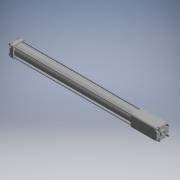
# Autodesk Inventor part: CE263-800(0)_BODY
Saved by Autodesk Inventor 2017.3 (Build 213256000, 256)
## iProperties
Part Number: CE263-800(0)_BODY
Material: Generic
Catalog Web Link: www.cadenas.de
Description: CE2 BODY-Stroke Reading Cylinder with Brake
Vendor: SMC
Document SubType Name: Modeling
Designer: partserver
Manufacturer: SMC
Mass: 2570.06 g
Surface Area: 5697.47 cm^2
Volume: 2570.06 cm^3
Density: 1 g/cm^3
Appearance: PSOLRGB-192-192-192
Category: PARTsolutions
Company: SMC
Title: CE263-800_BODY
Author: Cadenas PARTsolutions
Comments: Stroke Reading Cylinder with Brake
PSOL_IDENT_0: {$CADENAS_DATA\23d-libs\smc_jp\actuator\stroke_reading_cylinders\ce2\parts\ce2_body.prj},202 {VTYP=3
PSOL_IDENT_1: D},{NB=CE263-800(0)_BODY},{LINA=CE263-800_BODY},{NN=CE2 BODY},{DATE=05.07.2021 01:49:16},{GEOMDATE=2
PSOL_IDENT_2: 7.03.2020 05:40:07},{VERSION=},{LINEID=150},{WBVAR=THREAD1,STROKE,THREAD2},{WBNUMERIC=STROKE}  {NB=C
PSOL_IDENT_3: E263-800(0)_BODY},{LINA=CE263-800_BODY},{KT=DUMMY},{ORDER=CE263-800},{BORE=63},{THREAD1=},{STROKE=80
PSOL_IDENT_4: 0},{THREAD2=0},{A=35.000},{AA=60.000},{AL=32.000},{BB=98.500},{BL=27.000},{B=85.000},{C=48.500},{CC=
PSOL_IDENT_5: 23.000},{C1=64.000},{DD=24.000},{D=20.000},{EF=28.500},{EE=13.500},{E=40.000},{F=10.000},{FF=15.000}
PSOL_IDENT_6: ,{GA=174.000},{GB=17.000},{GC=26.000},{GD=67.000},{GL=18.000},{H1=11.000},{J=M10x1.25},{JRA=10.000},
PSOL_IDENT_7: {JRP=1.250},{K=9.000},{M=14.000},{MM=M18x1.5},{MMRA=18.000},{N=31.000},{NN=187.000},{P=3/8},{PND=16.
PSOL_IDENT_8: 662},{PH=11.700},{S=254.000},{W=0.000},{L1=22.000},{L2=73.000},{L3=72.000},{L4=9.100},{L5=5.300},{L6=
PSOL_IDENT_9: 35.000},{L7=13.000},{L8=9.500},{L9=14.000},{L10=9.200},{L11=9.200},{L12=2.500},{L13=9.000},{L14=48.5
PSOL_IDENT_10: 00},{L15=60.000},{LL1=23.000},{LL2=5.000},{LL3=6.000},{LL4=15.000},{LL5=8.000},{LL6=5.130},{LL7=4.50
PSOL_IDENT_11: 0},{LL8=38.500},{LL9=12.500},{LL0=109.500},{LL10=28.500},{L16=4.300},{L17=6.000},{L18=10.600},{L19=9
PSOL_IDENT_12: .820},{L20=10.500},{ZT=263.000},{H=58.000},{OFFET=18},{FONT=9}
NB: CE263-800(0)_BODY
NN: 187
NT: Stroke Reading Cylinder with Brake
NBSYN: $ORDER.($THREAD2.)_BODY
LINA: CE263-800_BODY
CATALOG: SMC (JP
BORE: 63
THREAD1: (-) Rc
STROKE: 800
THREAD2: on
A: 35
AA: 60
AL: 32
BB: 98.5
BL: 27
B: 85
C: 48.5
CC: 23
C1: 64
DD: 24
D: 20
EF: 28.5
EE: 13.5
E: 40
F: 10
FF: 15
GA: 174
GB: 17
GC: 26
GD: 67
GL: 18
H1: 11
J: M10x1.25
JRA: 10
JRP: 1.25
K: 9
M: 14
MM: M18x1.5
MMRA: 18
N: 31
P: 3/8
PND: 16.662
PH: 11.7
S: 254
W: 0
L1: 22
L2: 73
L3: 72
L4: 9.1
L5: 5.3
L6: 35
L7: 13
L8: 9.5
L9: 14
L10: 9.2
L11: 9.2
L12: 2.5
L13: 9
L14: 48.5
L15: 60
LL1: 23
LL2: 5
LL3: 6
LL4: 15
LL5: 8
LL6: 5.13
LL7: 4.5
LL8: 38.5
LL9: 12.5
LL0: 109.5
LL10: 28.5
L16: 4.3
L17: 6
L18: 10.6
L19: 9.82
L20: 10.5
ZT: 263
H: 58
SUPPLIER: SMC
ARTICLENO: CE263-800(0)_BODY
BOMINFO: CE263-800_BODY
CREATOR: CADENAS GmbH
Autodesk Inventor part; units mm, degrees
sketch "Sketch_1" plane through (0, 0, 0) normal (1, 0, 0) x (0, 1, 0)
  line L0 (31.5, 42.5) -> (-31.5, 42.5)
  arc A0 (-31.5, 42.5) -> (-42.5, 31.5) centre (-31.5, 31.5) ccw
  line L1 (-42.5, 31.5) -> (-42.5, -31.5)
  arc A1 (-42.5, -31.5) -> (-31.5, -42.5) centre (-31.5, -31.5) ccw
  line L2 (-31.5, -42.5) -> (31.5, -42.5)
  arc A2 (31.5, -42.5) -> (42.5, -31.5) centre (31.5, -31.5) ccw
  line L3 (42.5, -31.5) -> (42.5, 31.5)
  arc A3 (42.5, 31.5) -> (31.5, 42.5) centre (31.5, 31.5) ccw
  constraints: 8 end point, 8 point on circle, 4 centre point
extrude "Extrusion1" add sketch "Sketch_1" along normal blind 185.4
sketch "Sketch_2" plane through (0, 0, 0) normal (0, 0, 1) x (1, 0, 0)
  line L0 (187, 0) -> (185.4, 0)
  line L1 (185.4, 0) -> (185.4, 36.5)
  line L2 (185.4, 36.5) -> (187, 36.5)
  line L3 (187, 36.5) -> (187, 0)
  line L4 (187, 0) -> (185.4, 0)
  constraints: 10 end point
revolve "Revolution1" add sketch "Sketch_2" angle 360 about axis through (187, 0, 0) along (1, 0, 0)
sketch "Sketch_3" plane through (0, 0, 0) normal (0, 0, 1) x (1, 0, 0)
  line L0 (1023, 0) -> (187, 0)
  line L1 (187, 0) -> (187, 36)
  line L2 (187, 36) -> (1023, 36)
  line L3 (1023, 36) -> (1023, 0)
  line L4 (1023, 0) -> (187, 0)
  constraints: 10 end point
revolve "Revolution2" add sketch "Sketch_3" angle 360 about axis through (1023, 0, 0) along (1, 0, 0)
sketch "Sketch_41" plane through (0, 0, 0) normal (0, 0, 1) x (1, 0, 0)
  line L0 (1028.3, 0) -> (1023, 0)
  line L1 (1023, 0) -> (1023, 36.5)
  line L2 (1023, 36.5) -> (1028.3, 36.5)
  line L3 (1028.3, 36.5) -> (1028.3, 0)
  line L4 (1028.3, 0) -> (1023, 0)
  constraints: 10 end point
revolve "Revolution3" add sketch "Sketch_41" angle 360 about axis through (1028.3, 0, 0) along (1, 0, 0)
sketch "Sketch_4" plane through (1028.3, 0, 0) normal (1, 0, 0) x (0, 0, -1)
  line L0 (-42.5, 31.5) -> (-42.5, -31.5)
  arc A0 (-42.5, -31.5) -> (-31.5, -42.5) centre (-31.5, -31.5) ccw
  line L1 (-31.5, -42.5) -> (31.5, -42.5)
  arc A1 (31.5, -42.5) -> (42.5, -31.5) centre (31.5, -31.5) ccw
  line L2 (42.5, -31.5) -> (42.5, 31.5)
  arc A2 (42.5, 31.5) -> (31.5, 42.5) centre (31.5, 31.5) ccw
  line L3 (31.5, 42.5) -> (-31.5, 42.5)
  arc A3 (-31.5, 42.5) -> (-42.5, 31.5) centre (-31.5, 31.5) ccw
  constraints: 8 end point, 8 point on circle, 4 centre point
extrude "Extrusion2" add sketch "Sketch_4" along normal blind 25.7
sketch "Sketch_5" plane through (0, 42.5, 0) normal (0, 1, 0) x (1, 0, 0)
  line L0 (1024, 17.5) -> (1024, -17.5)
  line L1 (1024, -17.5) -> (1028.3, -19.9826)
  line L2 (1028.3, -19.9826) -> (1028.3, 19.9826)
  line L3 (1028.3, 19.9826) -> (1024, 17.5)
  constraints: 8 end point
extrude "Extrusion3" add sketch "Sketch_5" against normal blind 42.5
sketch "Sketch_11" plane through (0, 0, 0) normal (1, 0, 0) x (0, 1, 0)
  line L0 (-44.5, 44.5) -> (-44.5, -44.5)
  line L1 (-44.5, -44.5) -> (44.5, -44.5)
  line L2 (44.5, -44.5) -> (44.5, 44.5)
  line L3 (44.5, 44.5) -> (-44.5, 44.5)
  line L4 (23.5, 42.5) -> (-23.5, 42.5)
  line L5 (-23.5, 42.5) -> (-23.5, 40.4705)
  arc A0 (-40.4705, 23.5) -> (-23.5, 40.4705) centre (-32, 32) ccw
  line L6 (-40.4705, 23.5) -> (-42.5, 23.5)
  line L7 (-42.5, 23.5) -> (-42.5, -23.5)
  line L8 (-42.5, -23.5) -> (-40.4705, -23.5)
  arc A1 (-23.5, -40.4705) -> (-40.4705, -23.5) centre (-32, -32) ccw
  line L9 (-23.5, -40.4705) -> (-23.5, -42.5)
  line L10 (-23.5, -42.5) -> (23.5, -42.5)
  line L11 (23.5, -42.5) -> (23.5, -40.4705)
  arc A2 (40.4705, -23.5) -> (23.5, -40.4705) centre (32, -32) ccw
  line L12 (40.4705, -23.5) -> (42.5, -23.5)
  line L13 (42.5, -23.5) -> (42.5, 23.5)
  line L14 (42.5, 23.5) -> (40.4705, 23.5)
  arc A3 (23.5, 40.4705) -> (40.4705, 23.5) centre (32, 32) ccw
  line L15 (23.5, 40.4705) -> (23.5, 42.5)
  constraints: 32 end point, 8 point on circle, 4 centre point
extrude "Extrusion4" cut sketch "Sketch_11" along normal blind 9.5
sketch "Sketch_25" plane through (1054, 0, 0) normal (1, 0, 0) x (0, 0, -1)
  circle A0 centre (0, 0) radius 20
  constraints: 1 centre point
extrude "Extrusion5" add sketch "Sketch_25" along normal blind 6
sketch "Sketch_9" plane through (1054, 0, 0) normal (1, 0, 0) x (0, 0, -1)
  line L0 (-44.5, -44.5) -> (44.5, -44.5)
  line L1 (44.5, -44.5) -> (44.5, 44.5)
  line L2 (44.5, 44.5) -> (-44.5, 44.5)
  line L3 (-44.5, 44.5) -> (-44.5, -44.5)
  line L4 (-42.5, 23.5) -> (-42.5, -23.5)
  line L5 (-42.5, -23.5) -> (-40.4705, -23.5)
  arc A0 (-23.5, -40.4705) -> (-40.4705, -23.5) centre (-32, -32) ccw
  line L6 (-23.5, -40.4705) -> (-23.5, -42.5)
  line L7 (-23.5, -42.5) -> (23.5, -42.5)
  line L8 (23.5, -42.5) -> (23.5, -40.4705)
  arc A1 (40.4705, -23.5) -> (23.5, -40.4705) centre (32, -32) ccw
  line L9 (40.4705, -23.5) -> (42.5, -23.5)
  line L10 (42.5, -23.5) -> (42.5, 23.5)
  line L11 (42.5, 23.5) -> (40.4705, 23.5)
  arc A2 (23.5, 40.4705) -> (40.4705, 23.5) centre (32, 32) ccw
  line L12 (23.5, 40.4705) -> (23.5, 42.5)
  line L13 (23.5, 42.5) -> (-23.5, 42.5)
  line L14 (-23.5, 42.5) -> (-23.5, 40.4705)
  arc A3 (-40.4705, 23.5) -> (-23.5, 40.4705) centre (-32, 32) ccw
  line L15 (-40.4705, 23.5) -> (-42.5, 23.5)
  constraints: 32 end point, 8 point on circle, 4 centre point
extrude "Extrusion6" cut sketch "Sketch_9" against normal blind 10.6
sketch "Sketch_6" plane through (0, 32, 0) normal (0, 1, 0) x (1, 0, 0)
  line L0 (1068, 32) -> (-14, 32)
  line L1 (-14, 32) -> (-14, 36.233)
  line L2 (-14, 36.233) -> (-13.233, 37)
  line L3 (-13.233, 37) -> (4.5, 37)
  line L4 (4.5, 37) -> (4.5, 36.55)
  line L5 (4.5, 36.55) -> (1048.4, 36.55)
  line L6 (1048.4, 36.55) -> (1048.4, 37)
  line L7 (1048.4, 37) -> (1067.233, 37)
  line L8 (1067.233, 37) -> (1068, 36.233)
  line L9 (1068, 36.233) -> (1068, 32)
  line L10 (1068, 32) -> (-14, 32)
  constraints: 22 end point
revolve "Revolution4" add sketch "Sketch_6" angle 360 about axis through (1068, 32, -32) along (1, 0, 0)
thread "Thread1" size "M10x1.25" class "6g" standard "ISO Metric profile" full length
thread "Thread2" size "M10x1.25" class "6g" standard "ISO Metric profile" full length
pattern_linear "Rectangular Pattern1" count 2 spacing 64 along (0, 0, 1) count 2 spacing 64 along (0, -1, 0) of "Revolution4"
sketch "Sketch_8" plane through (0, 0, 0) normal (1, 0, 0) x (0, 1, 0)
  circle A0 centre (0, 0) radius 20
  constraints: 1 centre point
extrude "Extrusion7" add sketch "Sketch_8" against normal blind 10
sketch "Sketch_10" plane through (9.5, 0, 0) normal (1, 0, 0) x (0, 0, -1)
  circle A0 centre (-32, 32) radius 9.2
  constraints: 1 centre point
extrude "Extrusion8" add sketch "Sketch_10" against normal blind 2.5
pattern_linear "Rectangular Pattern2" count 2 spacing 64 along (0, 0, -1) count 2 spacing 64 along (0, -1, 0) of "Extrusion8"
sketch "Sketch_13" plane through (9.5, 0, 0) normal (1, 0, 0) x (0, 0, -1)
  line L0 (-38.5, 28.2472) -> (-32, 24.4944)
  line L1 (-32, 24.4944) -> (-25.5, 28.2472)
  line L2 (-25.5, 28.2472) -> (-25.5, 35.7528)
  line L3 (-25.5, 35.7528) -> (-32, 39.5056)
  line L4 (-32, 39.5056) -> (-38.5, 35.7528)
  line L5 (-38.5, 35.7528) -> (-38.5, 28.2472)
  constraints: 12 end point
extrude "Extrusion9" add sketch "Sketch_13" against normal blind 9
pattern_linear "Rectangular Pattern3" count 2 spacing 64 along (0, 0, -1) count 2 spacing 64 along (0, -1, 0) of "Extrusion9"
sketch "Sketch_15" plane through (1045.9, 0, 0) normal (1, 0, 0) x (0, 0, -1)
  line L0 (-40.5044, 27.09) -> (-32, 22.18)
  line L1 (-32, 22.18) -> (-23.4956, 27.09)
  line L2 (-23.4956, 27.09) -> (-23.4956, 36.91)
  line L3 (-23.4956, 36.91) -> (-32, 41.82)
  line L4 (-32, 41.82) -> (-40.5044, 36.91)
  line L5 (-40.5044, 36.91) -> (-40.5044, 27.09)
  constraints: 12 end point
extrude "Extrusion10" add sketch "Sketch_15" along normal blind 8
pattern_linear "Rectangular Pattern4" count 2 spacing 64 along (0, 0, -1) count 2 spacing 64 along (0, -1, 0) of "Extrusion10"
sketch "Sketch_17" plane through (1045.9, 0, 0) normal (1, 0, 0) x (0, 0, -1)
  circle A0 centre (-32, 32) radius 9.2
  constraints: 1 centre point
extrude "Extrusion11" add sketch "Sketch_17" against normal blind 2.5
pattern_linear "Rectangular Pattern5" count 2 spacing 64 along (0, 0, -1) count 2 spacing 64 along (0, -1, 0) of "Extrusion11"
sketch "Sketch_19" plane through (0, 42.5, 0) normal (0, 1, 0) x (1, 0, 0)
  line L0 (47.5, -10) -> (48.5, -10.4663)
  line L1 (48.5, -10.4663) -> (48.5, -30)
  line L2 (48.5, -30) -> (71.5, -30)
  line L3 (71.5, -30) -> (71.5, -10.4663)
  line L4 (71.5, -10.4663) -> (72.5, -10)
  line L5 (72.5, -10) -> (71.5, -9.5337)
  line L6 (71.5, -9.5337) -> (71.5, 30)
  line L7 (71.5, 30) -> (48.5, 30)
  line L8 (48.5, 30) -> (48.5, -9.5337)
  line L9 (48.5, -9.5337) -> (47.5, -10)
  constraints: 20 end point
extrude "Extrusion12" add sketch "Sketch_19" along normal blind 5
sketch "Sketch_20" plane through (0, 0, -6) normal (0, 0, 1) x (1, 0, 0)
  line L0 (48.5, 47.5) -> (71.5, 47.5)
  line L1 (71.5, 47.5) -> (70.3054, 56)
  line L2 (70.3054, 56) -> (49.6946, 56)
  line L3 (49.6946, 56) -> (48.5, 47.5)
  constraints: 8 end point
extrude "Extrusion13" add sketch "Sketch_20" against normal blind 15
sketch "Sketch_21" plane through (48.5, 47.5, 30) normal (0, 1, 0) x (1, 0, 0)
  circle A0 centre (11.5, 4.5) radius 4
  constraints: 1 centre point
extrude "Extrusion14" add sketch "Sketch_21" along normal blind 5.13
sketch "Sketch_22" plane through (48.5, 47.5, 30) normal (0, 1, 0) x (1, 0, 0)
  circle A0 centre (11.5, 55.5) radius 4
  constraints: 1 centre point
extrude "Extrusion15" add sketch "Sketch_22" along normal blind 5.13
sketch "Sketch_42" plane through (187, 0, 0) normal (1, 0, 0) x (0, 0, -1)
  line L0 (-16.3, 42.5) -> (-16.3, 38.5)
  arc A0 (-16.3, 38.5) -> (-8.7, 38.5) centre (-12.5, 38.5) ccw
  line L1 (-8.7, 38.5) -> (-8.7, 42.5)
  line L2 (-8.7, 42.5) -> (-16.3, 42.5)
  constraints: 6 end point, 2 point on circle, 1 centre point
extrude "Extrusion16" cut sketch "Sketch_42" against normal blind 28.5
sketch "Sketch_24" plane through (0, 38.5, 0) normal (0, 1, 0) x (1, 0, 0)
  line L0 (191, -12.5) -> (158.5, -12.5)
  line L1 (158.5, -12.5) -> (158.5, -9)
  line L2 (158.5, -9) -> (191, -9)
  line L3 (191, -9) -> (191, -12.5)
  line L4 (191, -12.5) -> (158.5, -12.5)
  constraints: 10 end point
revolve "Revolution5" add sketch "Sketch_24" angle 360 about axis through (191, 38.5, 12.5) along (1, 0, 0)
sketch "Sketch_23" plane through (0, 0, 42.5) normal (0, 0, 1) x (1, 0, 0)
  line L0 (166.4944, 0) -> (170.2472, -6.5)
  line L1 (170.2472, -6.5) -> (177.7528, -6.5)
  line L2 (177.7528, -6.5) -> (181.5056, 0)
  line L3 (181.5056, 0) -> (177.7528, 6.5)
  line L4 (177.7528, 6.5) -> (170.2472, 6.5)
  line L5 (170.2472, 6.5) -> (166.4944, 0)
  constraints: 12 end point
extrude "Extrusion17" add sketch "Sketch_23" along normal blind 5
sketch "Sketch_26" plane through (0, 0, 42.5) normal (0, 0, 1) x (1, 0, 0)
  circle A0 centre (174, 0) radius 4
  constraints: 1 centre point
extrude "Extrusion18" add sketch "Sketch_26" along normal blind 7.38
sketch "Sketch_27" plane through (0, 0, 42.5) normal (0, 0, 1) x (1, 0, 0)
  line L0 (1029.4944, 0) -> (1033.2472, -6.5)
  line L1 (1033.2472, -6.5) -> (1040.7528, -6.5)
  line L2 (1040.7528, -6.5) -> (1044.5056, 0)
  line L3 (1044.5056, 0) -> (1040.7528, 6.5)
  line L4 (1040.7528, 6.5) -> (1033.2472, 6.5)
  line L5 (1033.2472, 6.5) -> (1029.4944, 0)
  constraints: 12 end point
extrude "Extrusion19" add sketch "Sketch_27" along normal blind 5
sketch "Sketch_28" plane through (0, 0, 42.5) normal (0, 0, 1) x (1, 0, 0)
  circle A0 centre (1037, 0) radius 4
  constraints: 1 centre point
extrude "Extrusion20" add sketch "Sketch_28" along normal blind 7.38
sketch "Sketch_29" plane through (0, 0, 0) normal (0, 0, 1) x (1, 0, 0)
  line L0 (1037, 26.4843) -> (1037, 42.5)
  line L1 (1037, 42.5) -> (1045.331, 42.5)
  line L2 (1045.331, 42.5) -> (1044.475, 41.644)
  line L3 (1044.475, 41.644) -> (1044.475, 30.8)
  line L4 (1044.475, 30.8) -> (1037, 26.4843)
  line L5 (1037, 26.4843) -> (1037, 42.5)
  constraints: 12 end point
revolve "Revolution6" cut sketch "Sketch_29" angle 360 about axis through (1037, 26.4843, 0) along (0, -1, 0)
thread "Thread3" size "G16.662x1.337" designation "G 3/8" standard "ISO Pipe Threads" full length
sketch "Sketch_30" plane through (0, 0, -15) normal (0, 0, 1) x (1, 0, 0)
  line L0 (174, 26.4843) -> (174, 42.5)
  line L1 (174, 42.5) -> (182.331, 42.5)
  line L2 (182.331, 42.5) -> (181.475, 41.644)
  line L3 (181.475, 41.644) -> (181.475, 30.8)
  line L4 (181.475, 30.8) -> (174, 26.4843)
  line L5 (174, 26.4843) -> (174, 42.5)
  constraints: 12 end point
revolve "Revolution7" cut sketch "Sketch_30" angle 360 about axis through (174, 26.4843, -15) along (0, -1, 0)
thread "Thread4" size "G16.662x1.337" designation "G 3/8" standard "ISO Pipe Threads" full length
sketch "Sketch_31" plane through (0, 0, 18) normal (0, 0, 1) x (1, 0, 0)
  line L0 (93, 27.7961) -> (93, 42.5)
  line L1 (93, 42.5) -> (99.5785, 42.5)
  line L2 (99.5785, 42.5) -> (98.7225, 41.644)
  line L3 (98.7225, 41.644) -> (98.7225, 31.1)
  line L4 (98.7225, 31.1) -> (93, 27.7961)
  line L5 (93, 27.7961) -> (93, 42.5)
  constraints: 12 end point
revolve "Revolution8" cut sketch "Sketch_31" angle 360 about axis through (93, 27.7961, 18) along (0, -1, 0)
thread "Thread5" size "G13.157x1.337" designation "G 1/4" standard "ISO Pipe Threads" full length
sketch "Sketch_32" plane through (0, 0, 18) normal (0, 0, 1) x (1, 0, 0)
  line L0 (26, 27.7961) -> (26, 42.5)
  line L1 (26, 42.5) -> (32.5785, 42.5)
  line L2 (32.5785, 42.5) -> (31.7225, 41.644)
  line L3 (31.7225, 41.644) -> (31.7225, 31.1)
  line L4 (31.7225, 31.1) -> (26, 27.7961)
  line L5 (26, 27.7961) -> (26, 42.5)
  constraints: 12 end point
revolve "Revolution9" cut sketch "Sketch_32" angle 360 about axis through (26, 27.7961, 18) along (0, -1, 0)
thread "Thread6" size "G13.157x1.337" designation "G 1/4" standard "ISO Pipe Threads" full length
sketch "Sketch_33" plane through (0, 0, 0) normal (0, 0, 1) x (1, 0, 0)
  line L0 (1002, 0) -> (-10, 0)
  line L1 (-10, 0) -> (-10, 10)
  line L2 (-10, 10) -> (187, 10)
  line L3 (187, 10) -> (187, 31.5)
  line L4 (187, 31.5) -> (1002, 31.5)
  line L5 (1002, 31.5) -> (1002, 0)
  line L6 (1002, 0) -> (-10, 0)
  constraints: 14 end point
revolve "Revolution10" cut sketch "Sketch_33" angle 360 about axis through (1002, 0, 0) along (1, 0, 0)
sketch "Sketch_43" plane through (0, 42.5, 0) normal (0, 1, 0) x (1, 0, 0)
  line L0 (109.5, 20) -> (109.5, -24)
  line L1 (109.5, -24) -> (158.5, -24)
  line L2 (158.5, -24) -> (158.5, 20)
  line L3 (158.5, 20) -> (109.5, 20)
  constraints: 8 end point
extrude "Extrusion21" cut sketch "Sketch_43" against normal blind 0.5
ref_plane "N_XY" through (1023, 0, 0) normal (0, 0, 1) x (1, 0, 0)
ref_plane "N_YZ" through (1023, 0, 0) normal (1, 0, 0) x (0, 1, 0)
ref_plane "N_ZX" through (1023, 0, 0) normal (0, 1, 0) x (0, 0, 1)
ref_plane "body_XY" through (0, 0, 0) normal (-1, 0, 0) x (0, 0, -1)
ref_plane "body_YZ" through (0, 0, 0) normal (0, 0, -1) x (0, -1, 0)
ref_plane "body_ZX" through (0, 0, 0) normal (0, -1, 0) x (-1, 0, 0)
ref_plane "body_sw1_XY" through (187, 0, 0) normal (-1, 0, 0) x (0, 0, -1)
ref_plane "body_sw1_YZ" through (187, 0, 0) normal (0, 0, -1) x (0, -1, 0)
ref_plane "body_sw1_ZX" through (187, 0, 0) normal (0, -1, 0) x (-1, 0, 0)
ref_plane "body_sw2_XY" through (1023, 0, 0) normal (1, 0, 0) x (0, 0, -1)
ref_plane "body_sw2_YZ" through (1023, 0, 0) normal (0, 0, -1) x (0, 1, 0)
ref_plane "body_sw2_ZX" through (1023, 0, 0) normal (0, 1, 0) x (1, 0, 0)
ref_plane "body_trunnion_XY" through (605, 0, 0) normal (1, 0, 0) x (0, 0, -1)
ref_plane "body_trunnion_YZ" through (605, 0, 0) normal (0, 0, -1) x (0, 1, 0)
ref_plane "body_trunnion_ZX" through (605, 0, 0) normal (0, 1, 0) x (1, 0, 0)
ref_plane "body_head_XY" through (1054, 0, 0) normal (1, 0, 0) x (0, 0, -1)
ref_plane "body_head_YZ" through (1054, 0, 0) normal (0, 0, -1) x (0, 1, 0)
ref_plane "body_head_ZX" through (1054, 0, 0) normal (0, 1, 0) x (1, 0, 0)
body "Solid1"
